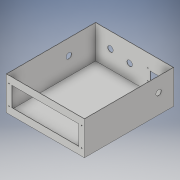
# Autodesk Inventor part: 18x12x6Box
Saved by Autodesk Inventor 2017 (Build 210142000, 142)
## iProperties
Created: 2017-02-28
Part Number: 18x12x6Box
Material: Generic
Document SubType Name: Modeling
Designer: Christer Hoeflinger
Density: 1 g/cm^3
Appearance: Default
Author: Christer Hoeflinger
Autodesk Inventor part; units mm, degrees
ref_plane "YZ Plane" through (0, 0, 0) normal (1, 0, 0) x (0, 1, 0)
ref_plane "XZ Plane" through (0, 0, 0) normal (0, 1, 0) x (-1, 0, 0)
ref_plane "XY Plane" through (0, 0, 0) normal (0, 0, 1) x (1, 0, 0)
sketch "Sketch1" plane through (0, 0, 0) normal (0, 1, 0) x (-1, 0, 0)
  line L0 (0, 0) -> (355.6, 0)
  line L1 (355.6, 0) -> (355.6, -406.4)
  line L2 (355.6, -406.4) -> (0, -406.4)
  line L3 (0, -406.4) -> (0, 0)
  dimension "d0" = 355.6
  dimension "d1" = 406.4
  constraints: 8 end point, 2 parallel, 1 horizontal, 1 perpendicular
  measures "d0" distance of L0.start L0.end
  measures "d1" distance of L2.end L0.start
extrude "Extrusion1" add sketch "Sketch1" along normal blind 152.4
sketch "Sketch2" plane through (0, 152.4, 0) normal (0, 1, 0) x (1, 0, 0)
  line L0 (-355.6, 0) -> (0, 0) projected
  line L1 (0, 0) -> (0, 406.4) projected
  line L2 (0, 406.4) -> (-355.6, 406.4) projected
  line L3 (-355.6, 406.4) -> (-355.6, 0) projected
  line L4 (-1.5875, 1.5875) -> (-354.0125, 1.5875)
  line L5 (-354.0125, 1.5875) -> (-354.0125, 404.8125)
  line L6 (-354.0125, 404.8125) -> (-1.5875, 404.8125)
  line L7 (-1.5875, 404.8125) -> (-1.5875, 1.5875)
  dimension "d4" = 1.5875
  dimension "d5" = 1.5875
  dimension "d6" = 1.5875
  dimension "d7" = 1.5875
  constraints: 8 end point, 2 parallel, 1 horizontal, 1 perpendicular
  measures "d4" distance between parallel lines of L0 L4
  measures "d5" distance between parallel lines of L2 L6
  measures "d6" distance between parallel lines of L1 L7
  measures "d7" distance between parallel lines of L3 L5
extrude "Extrusion2" cut sketch "Sketch2" against normal blind 150.8125 contours L4 L5 L6 L7
sketch "Sketch6" plane through (0, 0, 0) normal (1, 0, 0) x (0, 0, -1)
  line L0 (406.4, 0) -> (406.4, 152.4) projected
  line L1 (406.4, 0) -> (0, 0) projected
  circle A0 centre (337.3628, 87.884) radius 12.7
  dimension "d39" = 25.4
  dimension "d40" = 69.0372
  dimension "d41" = 87.884
  constraints: 1 centre point
  measures "d39" diameter of A0
  measures "d40" distance from line of A0.centre L0
  measures "d41" distance from line of L1 A0.centre
extrude "Extrusion4" cut sketch "Sketch6" against normal up to surface (1.5875 mm away)
sketch "Sketch7" plane through (0, 0, -406.4) normal (0, 0, -1) x (-1, 0, 0)
  circle A0 centre (286.5628, 82.804) radius 12.7
  line L0 (355.6, 0) -> (0, 0) projected
  line L1 (0, 0) -> (0, 152.4) projected
  circle A1 centre (199.136, 69.85) radius 12.7
  line L2 (1.5875, 152.4) -> (1.5875, 1.5875) projected
  line L3 (355.6, 0) -> (355.6, 152.4) projected
  point P0 (1.5875, 0)
  dimension "d23" = 82.804
  dimension "d25" = 25.4
  dimension "d28" = 25.4
  dimension "d128" = 199.136
  dimension "d129" = 69.0372
  dimension "d154" = 69.85
  constraints: 2 centre point
  measures "d23" distance from line of A0.centre L0
  measures "d25" diameter of A0
  measures "d28" diameter of A1
  measures "d128" distance from line of A1.centre L1
  measures "d129" distance from line of A0.centre L3
  measures "d154" distance from line of A1.centre L0
extrude "Extrusion5" cut sketch "Sketch7" against normal blind 25.4
sketch "Sketch9" plane through (-355.6, 0, 0) normal (0, 0, 1) x (1, 0, 0)
  line L0 (25.4, 31.75) -> (330.2, 31.75)
  line L1 (330.2, 31.75) -> (330.2, 120.65)
  line L2 (330.2, 120.65) -> (25.4, 120.65)
  line L3 (25.4, 120.65) -> (25.4, 31.75)
  line L4 (355.6, 0) -> (355.6, 152.4) projected
  line L5 (355.6, 0) -> (0, 0) projected
  line L6 (0, 0) -> (0, 152.4) projected
  dimension "d61" = 304.8
  dimension "d62" = 88.9
  dimension "d64" = 31.75
  dimension "d110" = 355.6
  dimension "d111" = 25.4
  constraints: 8 end point, 2 parallel, 1 horizontal, 1 perpendicular
  measures "d61" distance of L1.end L2.end
  measures "d62" distance of L0.end L1.end
  measures "d64" distance between parallel lines of L5 L0
  measures "d110" distance between parallel lines of L4 L6
  measures "d111" distance between parallel lines of L4 L1
extrude "Extrusion6" cut sketch "Sketch9" against normal blind 25.4
sketch "Sketch12" plane through (0, 0, -406.4) normal (0, 0, -1) x (-1, 0, 0)
  line L0 (50.8, 50.8) -> (105.918, 50.8)
  line L1 (105.918, 50.8) -> (105.918, 86.36)
  line L2 (105.918, 86.36) -> (50.8, 86.36)
  line L3 (50.8, 86.36) -> (50.8, 50.8)
  line L4 (63.7794, 81.9658) -> (92.9132, 81.9658) projected
  line L5 (0, 0) -> (0, 152.4) projected
  line L6 (355.6, 0) -> (0, 0) projected
  dimension "d120" = 35.56
  dimension "d121" = 55.118
  dimension "d122" = 50.8
  dimension "d123" = 50.8
  constraints: 8 end point, 2 parallel, 1 horizontal, 1 perpendicular
  measures "d120" distance of L2.end L0.start
  measures "d121" distance of L0.start L0.end
  measures "d122" distance between parallel lines of L5 L3
  measures "d123" distance between parallel lines of L6 L0
extrude "Extrusion8" cut sketch "Sketch12" against normal blind 25.4
sketch "Sketch13" plane through (-355.6, 0, -406.4) normal (-1, 0, 0) x (0, 0, 1)
  circle A0 centre (123.0122, 82.804) radius 12.7
  circle A1 centre (69.0372, 87.884) radius 12.7 projected
  circle A2 centre (69.0372, 87.884) radius 12.7 projected
  line L0 (0, 0) -> (406.4, 0) projected
  line L1 (0, 0) -> (0, 152.4) projected
  line L2 (406.4, 152.4) -> (0, 152.4) projected
  line L3 (406.4, 0) -> (406.4, 152.4) projected
  dimension "d132" = 25.4
  dimension "d133" = 87.884
  dimension "d134" = 82.804
  dimension "d135" = 123.0122
  constraints: 1 centre point
  measures "d132" diameter of A0
  measures "d133" distance from line of A1.centre L0
  measures "d134" distance from line of A0.centre L0
  measures "d135" distance from line of L1 A0.centre
extrude "Extrusion9" cut sketch "Sketch13" against normal up to surface (1.5875 mm away) contours A0
sketch "Sketch14" plane through (-355.6, 0, 0) normal (0, 0, 1) x (1, 0, 0)
  circle A0 centre (342.9, 120.65) radius 2.0828 projected
  circle A1 centre (342.9, 31.75) radius 2.0828 projected
  circle A2 centre (12.7, 31.75) radius 2.0828 projected
  circle A3 centre (12.7, 120.65) radius 2.0828 projected
  point P0 (355.6, 0)
  constraints: 4 coincident
hole "Hole1" at (-12.7, 120.65, 0) at (-12.7, 31.75, 0) at (-342.9, 31.75, 0) at (-342.9, 120.65, 0) direction (0, 0, -1) diameter 4.1656 depth 6.35 tip angle 118
sketch "Sketch15" plane through (0, 0, -406.4) normal (0, 0, -1) x (-1, 0, 0)
  circle A0 centre (40.64, 41.91) radius 1.7526 projected
  circle A1 centre (116.84, 92.71) radius 1.7526 projected
  circle A2 centre (40.64, 92.71) radius 1.7526 projected
  circle A3 centre (116.84, 41.91) radius 1.7526 projected
  circle A4 centre (56.261, 55.372) radius 2.1463 projected
  circle A5 centre (101.219, 79.248) radius 2.1463 projected
  circle A6 centre (101.219, 55.372) radius 2.1463 projected
  circle A7 centre (56.261, 79.248) radius 2.1463 projected
  arc A8 (64.1858, 79.0702) -> (57.8358, 72.7202) centre (64.1858, 72.7202) ccw projected
  line L0 (64.1858, 79.0702) -> (93.3196, 79.0702) projected
  arc A9 (99.6696, 72.7202) -> (93.3196, 79.0702) centre (93.3196, 72.7202) ccw projected
  line L1 (99.6696, 72.7202) -> (99.6696, 61.5442) projected
  arc A10 (93.3196, 55.1942) -> (99.6696, 61.5442) centre (93.3196, 61.5442) ccw projected
  line L2 (93.3196, 55.1942) -> (64.1858, 55.1942) projected
  arc A11 (57.8358, 61.5442) -> (64.1858, 55.1942) centre (64.1858, 61.5442) ccw projected
  line L3 (57.8358, 61.5442) -> (57.8358, 72.7202) projected
  line L4 (123.19, 99.06) -> (34.29, 99.06) projected
  line L5 (34.29, 99.06) -> (34.29, 35.56) projected
  line L6 (34.29, 35.56) -> (123.19, 35.56) projected
  line L7 (123.19, 35.56) -> (123.19, 99.06) projected
  line L8 (74.4123, 41.91) -> (73.7537, 41.91) projected
  line L9 (73.7537, 41.91) -> (73.7537, 47.6322) projected
  line L10 (73.7537, 47.6322) -> (72.6267, 47.6322) projected
  line L11 (72.6267, 47.6322) -> (72.6267, 48.2806) projected
  line L12 (72.6267, 48.2806) -> (75.7245, 48.2806) projected
  line L13 (75.7245, 48.2806) -> (75.7245, 47.6322) projected
  line L14 (75.7245, 47.6322) -> (74.5718, 47.6322) projected
  line L15 (74.5718, 47.6322) -> (74.5718, 43.3766) projected
  line L16 (74.5718, 43.3766) -> (75.7245, 43.3766) projected
  line L17 (75.7245, 43.3766) -> (75.7245, 42.7951) projected
  spline S0 degree 2 poles (75.7245, 42.7951) (75.071, 42.7951) (74.4535, 42.4246) (74.4123, 41.91) knots 0 0 0 1 2 2 2 projected
  line L18 (82.8979, 42.6047) -> (84.2409, 42.6047) projected
  line L19 (84.2409, 42.6047) -> (84.2409, 41.9306) projected
  line L20 (84.2409, 41.9306) -> (82.0539, 41.9306) projected
  line L21 (82.0539, 41.9306) -> (82.0539, 46.6288) projected
  spline S1 degree 2 poles (82.0539, 46.6288) (82.0539, 47.4624) (83.0728, 48.3681) (83.9322, 48.3681) knots 0 0 0 1 2 2 2 projected
  spline S2 degree 2 poles (83.9322, 48.3681) (84.138, 48.3681) (84.8224, 48.296) (85.054, 48.2446) knots 0 0 0 1 2 2 2 projected
  line L22 (85.054, 48.2446) -> (85.054, 47.4315) projected
  line L23 (85.054, 47.4315) -> (85.0077, 47.4315) projected
  spline S3 degree 2 poles (85.0077, 47.4315) (84.8327, 47.4933) (84.313, 47.6373) (84.0454, 47.6373) knots 0 0 0 1 2 2 2 projected
  spline S4 degree 2 poles (84.0454, 47.6373) (83.6543, 47.6373) (83.186, 47.4572) (83.078, 47.2926) knots 0 0 0 1 2 2 2 projected
  spline S5 degree 2 poles (83.078, 47.2926) (82.9596, 47.1228) (82.8979, 46.6288) (82.8979, 46.3046) knots 0 0 0 1 2 2 2 projected
  line L24 (82.8979, 46.3046) -> (82.8979, 42.6047) projected
  spline S6 degree 2 poles (80.4896, 42.7951) (79.8361, 42.7951) (79.2186, 42.4246) (79.1774, 41.91) knots 0 0 0 1 2 2 2 projected
  line L25 (79.1774, 41.91) -> (78.5187, 41.91) projected
  line L26 (78.5187, 41.91) -> (78.5187, 47.6322) projected
  line L27 (78.5187, 47.6322) -> (77.3918, 47.6322) projected
  line L28 (77.3918, 47.6322) -> (77.3918, 48.2806) projected
  line L29 (77.3918, 48.2806) -> (80.4896, 48.2806) projected
  line L30 (80.4896, 48.2806) -> (80.4896, 47.6322) projected
  line L31 (80.4896, 47.6322) -> (79.3369, 47.6322) projected
  line L32 (79.3369, 47.6322) -> (79.3369, 43.3766) projected
  line L33 (79.3369, 43.3766) -> (80.4896, 43.3766) projected
  line L34 (80.4896, 43.3766) -> (80.4896, 42.7951) projected
  point P0 (0, 0)
  constraints: 4 coincident
hole "Hole2" at (-116.84, 92.71, -406.4) at (-116.84, 41.91, -406.4) at (-40.64, 41.91, -406.4) at (-40.64, 92.71, -406.4) direction (0, 0, 1) diameter 4.1656 depth 6.35 tip angle 118
thread "Thread1" size "8-32 UNC" class "2B" standard "ANSI Unified Screw Threads" full length
thread "Thread2" size "8-32 UNC" class "2B" standard "ANSI Unified Screw Threads" full length
thread "Thread3" size "8-32 UNC" class "2B" standard "ANSI Unified Screw Threads" full length
thread "Thread4" size "8-32 UNC" class "2B" standard "ANSI Unified Screw Threads" full length
thread "Thread5" size "8-32 UNC" class "2B" standard "ANSI Unified Screw Threads" full length
thread "Thread6" size "8-32 UNC" class "2B" standard "ANSI Unified Screw Threads" full length
thread "Thread7" size "8-32 UNC" class "2B" standard "ANSI Unified Screw Threads" full length
thread "Thread8" size "8-32 UNC" class "2B" standard "ANSI Unified Screw Threads" full length
equation "\"d5\" = d4"
equation "\"d6\" = d4"
equation "\"d7\" = d4"
equation "\"d28\" = d25"
equation "\"d26\" = d28"
equation "\"d111\" = -0.5 * d61 + 0.5 * d110"
body "Solid1"
